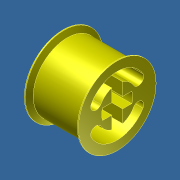
# Autodesk Inventor part: LEGO Brick 3482
Saved by Autodesk Inventor 2011 SP2 (Build 150553200, 553)
## iProperties
Company: Allseas Engineering BV
Created: 2011-11-30
Part Number: LEGO Brick 3482
Cost Center: 0 kg
Material: Steel
Document SubType Name: Modeling
Designer: BvH
Authority: 0 mm^3
Stock Number: =<Filenr>_<Document number>
Density: 7.85 g/cm^3
Mass: 5.27848 g
Surface Area: 11.2041 cm^2
Volume: 0.672418 cm^3
Act. Code: DW000
SaveDate: 2011-07-28
SaveTime: 18:32
FileName: Standard
TotalMass: 0 kg
TotalVolume: 0 mm^3
Subject: =<Title><TITLE 1_2> <TITLE 2_2>
Author: BvH
Autodesk Inventor part; units mm, degrees
ref_plane "YZ Plane" through (0, 0, 0) normal (1, 0, 0) x (0, 1, 0)
ref_plane "XZ Plane" through (0, 0, 0) normal (0, 1, 0) x (-1, 0, 0)
ref_plane "XY Plane" through (0, 0, 0) normal (0, 0, 1) x (1, 0, 0)
sketch "Sketch1" plane through (0, 0, 0) normal (0, 0, 1) x (1, 0, 0)
  line L0 (0, -1.5) -> (0, 9) construction
  line L1 (-4, 7.25) -> (-3.8557, 7.25)
  line L2 (-3.8557, 7.25) -> (-3.4226, 6.5)
  line L3 (-3.4226, 6.5) -> (3.4226, 6.5)
  line L4 (3.4226, 6.5) -> (3.8557, 7.25)
  line L5 (3.8557, 7.25) -> (4, 7.25)
  line L6 (4, 7.25) -> (4, 0)
  line L7 (4, 0) -> (-4, 0)
  line L8 (-4, 0) -> (-4, 7.25)
  point P0 (0, 0)
  point P1 (0, 6.5)
  point P2 (4, 7.5)
  dimension "d0" = 13
  dimension "d1" = 60
  dimension "d2" = 8
  dimension "d3" = 15
  dimension "d4" = 14.5
  constraints: 16 end point, 4 horizontal, 3 point on line, 2 equal length, 2 midpoint, 2 vertical
  measures "d0" diameter of L3 L7
  measures "d1" angle of L2 L3
  measures "d2" distance between parallel lines of L6 L8
  measures "d3" diameter of point (4, 7.5) L7
  measures "d4" diameter of L1 L7
revolve "Revolution1" add sketch "Sketch1" angle 360 about axis through (4, 0, 0) along (-1, 0, 0)
sketch "Sketch2" plane through (0, 0, 0) normal (1, 0, 0) x (0, 1, 0)
  circle A0 centre (0, 0) radius 2.3
  line L0 (0.8, 2.1564) -> (0.8, 0.8)
  line L1 (0.8, -0.8) -> (0.8, -2.1564)
  line L2 (-2.1564, 0.8) -> (-0.8, 0.8)
  line L3 (0.8, 0.8) -> (2.1564, 0.8)
  line L4 (2.1564, -0.8) -> (0.8, -0.8)
  line L5 (-0.8, -0.8) -> (-2.1564, -0.8)
  line L6 (-0.8, 2.1564) -> (-0.8, 0.8)
  line L7 (-0.8, -0.8) -> (-0.8, -2.1564)
  dimension "d6" = 4.6
  dimension "d7" = 1.6
  constraints: 16 end point, 7 equal length, 4 horizontal, 4 vertical, 1 coincident, 10 other
  measures "d7" distance between parallel lines of L0 L6
extrude "Extrusion1" cut sketch "Sketch2" along normal through all both and the other way through all contours A0 L4 L1 L7 L5 L2 L6 L0 L3
sketch "Sketch3" plane through (0, 0, 0) normal (1, 0, 0) x (0, 1, 0)
  circle A0 centre (0, 0) radius 2.3 construction
  arc A1 (3.2909, 1.9) -> (-3.2909, 1.9) centre (0, 0) ccw
  arc A2 (4.6765, 2.7) -> (-4.6765, 2.7) centre (0, 0) ccw
  arc A3 (-3.2909, -1.9) -> (3.2909, -1.9) centre (0, 0) ccw
  arc A4 (-4.6765, -2.7) -> (4.6765, -2.7) centre (0, 0) ccw
  arc A5 (3.2909, 1.9) -> (4.6765, 2.7) centre (3.9837, 2.3) ccw
  arc A6 (4.6765, -2.7) -> (3.2909, -1.9) centre (3.9837, -2.3) ccw
  arc A7 (-4.6765, 2.7) -> (-3.2909, 1.9) centre (-3.9837, 2.3) ccw
  arc A8 (-3.2909, -1.9) -> (-4.6765, -2.7) centre (-3.9837, -2.3) ccw
  line L0 (-3.9837, 2.3) -> (0, 0) construction
  line L1 (0, 0) -> (3.9837, 2.3) construction
  line L2 (3.9837, -2.3) -> (0, 0) construction
  line L3 (-3.9837, -2.3) -> (0, 0) construction
  line L4 (0, -6.16) -> (0, 6.16) construction
  line L5 (-5.8947, 0) -> (5.8947, 0) construction
  dimension "d10" = 1.6
  dimension "d11" = 120
  dimension "d12" = 120
  dimension "d15" = 3.8
  constraints: 16 point on circle, 8 centre point, 8 end point, 8 tangent, 4 coincident, 2 concentric, 2 other
  measures "d10" radial gap between concentric circles of A4 A3
  measures "d11" angle of L0 L1
  measures "d12" angle of L3 L2
  measures "d15" radius of A3
extrude "Extrusion2" cut sketch "Sketch3" along normal through all both and the other way through all
sketch "Sketch4" plane through (0, 0, 0) normal (1, 0, 0) x (0, 1, 0)
  arc A0 (3.2909, 1.9) -> (-3.2909, 1.9) centre (0, 0) ccw projected
  arc A1 (-3.2909, -1.9) -> (3.2909, -1.9) centre (0, 0) ccw projected
  line L0 (0.8, -0.8) -> (0.8, -2.1564) construction
  line L1 (-0.8, -2.1564) -> (-0.8, -0.8) construction
  line L2 (0.8, 3.7148) -> (0.8, -3.7148)
  line L3 (-0.8, 3.7148) -> (-0.8, -3.7148)
  constraints: 4 end point, 4 point on circle, 2 collinear, 2 vertical
extrude "Extrusion3" cut sketch "Sketch4" along normal through all both and the other way through all
body "Solid1"
